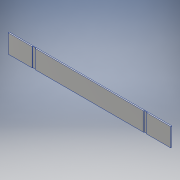
# Autodesk Inventor part: 앞판_밑
Saved by Autodesk Inventor 2017 (Build 210142000, 142)
## iProperties
Part Number: 앞판_밑
Material: 알루미늄 6061
Document SubType Name: Modeling
Designer: minom
Density: 2.7 g/cm^3
Appearance: 알루미늄 - 평지
Mass: 50.7514 g
Surface Area: 205.432 cm^2
Volume: 18.7968 cm^3
Author: minom
Autodesk Inventor part; units mm, degrees
ref_plane "YZ Plane" through (0, 0, 0) normal (1, 0, 0) x (0, 1, 0)
ref_plane "XZ Plane" through (0, 0, 0) normal (0, 1, 0) x (-1, 0, 0)
ref_plane "XY Plane" through (0, 0, 0) normal (0, 0, 1) x (1, 0, 0)
sketch "스케치1" plane through (0, 0, 0) normal (0, 1, 0) x (-1, 0, 0)
  line L0 (74, 43) -> (-216, 43)
  line L1 (-216, 43) -> (-216, 76)
  line L2 (-216, 76) -> (74, 76)
  line L3 (74, 76) -> (74, 43)
  point P0 (0, 0)
  dimension "d0" = 290
  dimension "d1" = 33
  constraints: 8 end point, 2 parallel, 1 horizontal, 1 perpendicular
  measures "d0" distance of L1.end L2.end
  measures "d1" distance of L0.end L1.end
extrude "돌출1" add sketch "스케치1" along normal blind 2
sketch "스케치2" plane through (0, 0, 0) normal (0, -1, 0) x (1, 0, 0)
  line L0 (216, 43) -> (-74, 43) projected
  line L1 (-74, 76) -> (216, 76) projected
  line L2 (173, 43) -> (167.8, 43)
  line L3 (167.8, 43) -> (167.8, 76)
  line L4 (167.8, 76) -> (173, 76)
  line L5 (173, 76) -> (173, 43)
  line L6 (216, 43) -> (216, 76) projected
  line L7 (216, 76) -> (-74, 76) projected
  line L8 (-74, 43) -> (216, 43) projected
  line L9 (-31, 76) -> (-25.8, 76)
  line L10 (-25.8, 76) -> (-25.8, 43)
  line L11 (-25.8, 43) -> (-31, 43)
  line L12 (-31, 43) -> (-31, 76)
  line L13 (-74, 76) -> (-74, 43) projected
  point P0 (0, 0)
  dimension "d4" = 5.2
  dimension "d5" = 43
  dimension "d6" = 5.2
  dimension "d7" = 43
  constraints: 16 end point, 4 parallel, 4 point on line, 2 horizontal, 2 perpendicular
  measures "d4" distance between parallel lines of L3 L5
  measures "d5" distance between parallel lines of L5 L6
  measures "d6" distance of L10.end L11.end
  measures "d7" distance between parallel lines of L12 L13
extrude "돌출2" cut sketch "스케치2" against normal blind 1 contours L0 L3 L1 L5 | L0 L12 L1 L10
